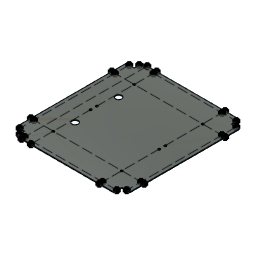
Hot Plate Mounting Plate (Autodesk Fusion 360 design; units mm, degrees)
Autodesk Fusion 360 part; units mm, degrees
sketch "Sketch1" plane through (0, 0, 0) normal (0, 0, 1) x (1, 0, 0) in component "Hot Plate Mounting Plate"
  line L0 (0, 0) -> (-182, 0) construction
  line L1 (-182, 0) -> (-182, -202) construction
  line L2 (-182, -202) -> (0, -202) construction
  line L3 (0, -202) -> (0, 0) construction
  line L4 (-91, -202) -> (-91, 0) construction
  line L5 (0, -101) -> (-182, -101) construction
  line L6 (-91, 0) -> (-13, 0)
  line L7 (-91, 0) -> (-169, 0)
  line L8 (-91, -202) -> (-13, -202)
  line L9 (-91, -202) -> (-169, -202)
  line L10 (0, -101) -> (0, -13)
  line L11 (0, -101) -> (0, -189)
  line L12 (-182, -101) -> (-182, -189)
  line L13 (-182, -101) -> (-182, -13)
  line L14 (-182, -13) -> (0, -13) construction
  line L15 (0, -189) -> (-182, -189) construction
  line L16 (-13, -202) -> (-13, 0) construction
  line L17 (-169, 0) -> (-169, -202) construction
  line L18 (0, -189) -> (-13, -189)
  line L19 (-13, -202) -> (-13, -189)
  line L20 (-169, -202) -> (-169, -189)
  line L21 (-182, -189) -> (-169, -189)
  line L22 (0, -13) -> (-13, -13)
  line L23 (-13, 0) -> (-13, -13)
  line L24 (-169, 0) -> (-169, -13)
  line L25 (-182, -13) -> (-169, -13)
  dimension "d1" = 182
  dimension "d2" = 202
  dimension "d3" = 78
  dimension "d4" = 78
  dimension "d5" = 78
  dimension "d6" = 78
  dimension "d7" = 88
  dimension "d8" = 88
  dimension "d9" = 88
  dimension "d10" = 88
  constraint horizontal L0
  constraint vertical L1
  constraint horizontal L2
  constraint vertical L3
  constraint coincident L0.start L3.end
  constraint midpoint L2 L4.start
  constraint midpoint L0 L4.end
  constraint midpoint L3 L5.start
  constraint midpoint L1 L5.end
  constraint perpendicular L4 L6
  constraint perpendicular L4 L7
  constraint perpendicular L4 L8
  constraint perpendicular L4 L9
  constraint perpendicular L5 L10
  constraint perpendicular L5 L11
  constraint perpendicular L5 L12
  constraint perpendicular L5 L13
  constraint coincident L15 L18.end
  constraint coincident L16 L18.end
  constraint coincident L15 L20.end
  constraint coincident L17 L20.end
  constraint coincident L14 L22.end
  constraint coincident L16 L22.end
  constraint coincident L14 L24.end
  constraint coincident L17 L24.end
  measures "d1" distance of L0.start L0.end
  measures "d2" distance of L0.start L2.end
  measures "d3" distance of L4.end L6.end
  measures "d4" distance of L4.end L7.end
  measures "d5" distance of L4.start L8.end
  measures "d6" distance of L4.start L9.end
  measures "d7" distance of L5.start L10.end
  measures "d8" distance of L5.start L11.end
  measures "d9" distance of L5.end L12.end
  measures "d10" distance of L5.end L13.end
extrude "Extrude1" add sketch "Sketch1" along normal blind 1 in component "Hot Plate Mounting Plate"
sketch "Sketch3" plane through (0, 0, 1) normal (0, 0, 1) x (-1, 0, 0) in component "Hot Plate Mounting Plate"
  line L0 (182, 13) -> (182, 189)
  line L1 (182, 189) -> (169, 189)
  line L2 (169, 189) -> (169, 202)
  line L3 (169, 202) -> (13, 202)
  line L4 (13, 202) -> (13, 189)
  line L5 (13, 189) -> (0, 189)
  line L6 (0, 189) -> (0, 13)
  line L7 (0, 13) -> (13, 13)
  line L8 (13, 13) -> (13, 0)
  line L9 (13, 0) -> (169, 0)
  line L10 (169, 0) -> (169, 13)
  line L11 (169, 13) -> (182, 13)
  line L12 (177, 13) -> (177, 189) construction
  line L13 (169, 5) -> (13, 5) construction
  line L14 (5, 13) -> (5, 189) construction
  line L15 (13, 197) -> (169, 197) construction
  line L16 (182, 36) -> (0, 36) construction
  line L17 (182, 166) -> (0, 166) construction
  line L18 (146, 0) -> (146, 202) construction
  line L19 (36, 0) -> (36, 202) construction
  circle A0 centre (146, 5) radius 1.75
  circle A1 centre (177, 36) radius 1.75
  circle A2 centre (177, 166) radius 1.75
  circle A3 centre (36, 197) radius 1.75
  circle A4 centre (5, 166) radius 1.75
  circle A5 centre (5, 36) radius 1.75
  circle A6 centre (36, 5) radius 1.75
  line L20 (161, 202) -> (161, 0) construction
  circle A7 centre (161, 197) radius 1.75
  dimension "d44" = 5
  dimension "d45" = 5
  dimension "d46" = 5
  dimension "d47" = 5
  dimension "d48" = 23
  dimension "d49" = 23
  dimension "d50" = 23
  dimension "d51" = 23
  dimension "d52" = 3.5
  dimension "d53" = 3.5
  dimension "d54" = 3.5
  dimension "d56" = 3.5
  dimension "d57" = 3.5
  dimension "d60" = 3.5
  dimension "d61" = 3.5
  dimension "d62" = 8
  dimension "d63" = 3.5
  constraint coincident L11 L12.start
  constraint coincident L1 L12.end
  constraint perpendicular L1 L12
  constraint coincident L10 L13.start
  constraint coincident L8 L13.end
  constraint perpendicular L8 L13
  constraint coincident L7 L14.start
  constraint coincident L5 L14.end
  constraint perpendicular L5 L14
  constraint coincident L4 L15.start
  constraint coincident L2 L15.end
  constraint perpendicular L2 L15
  constraint coincident L0 L16.start
  constraint coincident L6 L16.end
  constraint perpendicular L6 L16
  constraint coincident L0 L17.start
  constraint coincident L6 L17.end
  constraint perpendicular L6 L17
  constraint coincident L9 L18.start
  constraint perpendicular L9 L18
  constraint coincident L9 L19.start
  constraint coincident L3 L19.end
  constraint perpendicular L3 L19
  constraint coincident L13 A0.centre
  constraint coincident L18 A0.centre
  constraint coincident L16 A1.centre
  constraint coincident L12 A1.centre
  constraint coincident L17 A2.centre
  constraint coincident L12 A2.centre
  constraint coincident L3 L18.end
  constraint coincident L15 A3.centre
  constraint coincident L19 A3.centre
  constraint coincident L17 A4.centre
  constraint coincident L14 A4.centre
  constraint coincident L16 A5.centre
  constraint coincident L14 A5.centre
  constraint coincident L19 A6.centre
  constraint coincident L13 A6.centre
  constraint coincident L3 L20.start
  constraint coincident L9 L20.end
  constraint perpendicular L9 L20
  constraint coincident L15 A7.centre
  constraint coincident L20 A7.centre
  measures "d44" distance of L0 L12
  measures "d45" distance of L3 L15
  measures "d46" distance of L6 L14
  measures "d47" distance of L9 L13
  measures "d48" distance of L11 L16
  measures "d49" distance of L10 L18
  measures "d50" distance of L8 L19
  measures "d51" distance of L1 L17
  measures "d52" diameter of A0
  measures "d53" diameter of A1
  measures "d54" diameter of A2
  measures "d56" diameter of A3
  measures "d57" diameter of A4
  measures "d60" diameter of A5
  measures "d61" diameter of A6
  measures "d62" distance of L2 L20
  measures "d63" diameter of A7
extrude "Extrude3" cut sketch "Sketch3" against normal up to surface (1 mm away) contours A0 | A1 | A2 | A3 | A4 | A5 | A6 | A7 in component "Hot Plate Mounting Plate"
sketch "Sketch4" plane through (0, 0, 1) normal (0, 0, 1) x (-1, 0, 0) in component "Hot Plate Mounting Plate"
  circle A0 centre (5, 36) radius 1.75
  circle A1 centre (5, 166) radius 1.75
  circle A2 centre (177, 166) radius 1.75
  circle A3 centre (36, 5) radius 1.75
  circle A4 centre (146, 5) radius 1.75
  circle A5 centre (36, 197) radius 1.75
  circle A6 centre (177, 36) radius 1.75
  circle A7 centre (161, 197) radius 1.75
  line L0 (182, 13) -> (182, 189)
  line L1 (182, 189) -> (169, 189)
  line L2 (169, 189) -> (169, 202)
  line L3 (169, 202) -> (13, 202)
  line L4 (13, 202) -> (13, 189)
  line L5 (13, 189) -> (0, 189)
  line L6 (0, 189) -> (0, 13)
  line L7 (0, 13) -> (13, 13)
  line L8 (13, 13) -> (13, 0)
  line L9 (13, 0) -> (169, 0)
  line L10 (169, 0) -> (169, 13)
  line L11 (169, 13) -> (182, 13)
  line L12 (182, 101) -> (0, 101) construction
  line L13 (91, 0) -> (91, 202) construction
  line L14 (31, 31) -> (151, 31) construction
  line L15 (151, 31) -> (151, 171) construction
  line L16 (151, 171) -> (31, 171) construction
  line L17 (31, 171) -> (31, 31) construction
  line L18 (31, 31) -> (151, 171) construction
  line L19 (151, 31) -> (31, 171) construction
  line L20 (146, 31) -> (146, 171) construction
  line L21 (151, 36) -> (31, 36) construction
  line L22 (36, 31) -> (36, 171) construction
  line L23 (151, 166) -> (31, 166) construction
  circle A8 centre (146, 36) radius 1.75
  line L24 (151, 96) -> (31, 96) construction
  line L25 (151, 106) -> (31, 106) construction
  circle A9 centre (146, 96) radius 1.75
  circle A10 centre (36, 96) radius 1.75
  circle A11 centre (146, 106) radius 1.75
  circle A12 centre (36, 106) radius 1.75
  circle A13 centre (146, 166) radius 1.75
  circle A14 centre (36, 166) radius 1.75
  circle A15 centre (36, 36) radius 1.75
  line L26 (151, 66) -> (31, 66) construction
  line L27 (151, 136) -> (31, 136) construction
  line L28 (141, 31) -> (141, 171) construction
  circle A16 centre (141, 66) radius 5
  circle A17 centre (141, 136) radius 5
  point P0 (91, 101)
  dimension "d64" = 120
  dimension "d65" = 140
  dimension "d66" = 5
  dimension "d67" = 5
  dimension "d68" = 5
  dimension "d69" = 5
  dimension "d70" = 3.5
  dimension "d71" = 5
  dimension "d72" = 5
  dimension "d73" = 3.5
  dimension "d74" = 3.5
  dimension "d75" = 3.5
  dimension "d76" = 3.5
  dimension "d77" = 3.5
  dimension "d78" = 3.5
  dimension "d79" = 3.5
  dimension "d83" = 35
  dimension "d84" = 35
  dimension "d85" = 10
  dimension "d86" = 10
  dimension "d87" = 10
  constraint midpoint L0 L12.start
  constraint midpoint L6 L12.end
  constraint midpoint L9 L13.start
  constraint midpoint L3 L13.end
  constraint horizontal L14
  constraint perpendicular L14 L15
  constraint parallel L14 L16
  constraint parallel L15 L17
  constraint coincident L18 P0
  constraint coincident L19 P0
  constraint midpoint L12 P0
  constraint coincident L14 L20.start
  constraint coincident L16 L20.end
  constraint perpendicular L16 L20
  constraint coincident L15 L21.start
  constraint coincident L17 L21.end
  constraint perpendicular L17 L21
  constraint coincident L14 L22.start
  constraint coincident L16 L22.end
  constraint perpendicular L16 L22
  constraint coincident L15 L23.start
  constraint coincident L17 L23.end
  constraint perpendicular L17 L23
  constraint coincident L20 A8.centre
  constraint coincident L21 A8.centre
  constraint coincident L15 L24.start
  constraint coincident L17 L24.end
  constraint perpendicular L17 L24
  constraint coincident L15 L25.start
  constraint coincident L17 L25.end
  constraint perpendicular L17 L25
  constraint coincident L24 A9.centre
  constraint coincident L20 A9.centre
  constraint coincident L24 A10.centre
  constraint coincident L22 A10.centre
  constraint coincident L25 A11.centre
  constraint coincident L20 A11.centre
  constraint coincident L25 A12.centre
  constraint coincident L22 A12.centre
  constraint coincident L23 A13.centre
  constraint coincident L20 A13.centre
  constraint coincident L23 A14.centre
  constraint coincident L22 A14.centre
  constraint coincident L22 A15.centre
  constraint coincident L21 A15.centre
  constraint coincident L15 L26.start
  constraint coincident L17 L26.end
  constraint perpendicular L17 L26
  constraint coincident L15 L27.start
  constraint coincident L17 L27.end
  constraint perpendicular L17 L27
  constraint coincident L14 L28.start
  constraint coincident L16 L28.end
  constraint perpendicular L16 L28
  constraint coincident L26 A16.centre
  constraint coincident L28 A16.centre
  constraint coincident L27 A17.centre
  constraint coincident L28 A17.centre
  measures "d64" distance of L15.end L16.end
  measures "d65" distance of L14.end L15.end
  measures "d66" distance of L16 L23
  measures "d67" distance of L15 L20
  measures "d68" distance of L14 L21
  measures "d69" distance of L17 L22
  measures "d70" diameter of A8
  measures "d71" distance of L12 L24
  measures "d72" distance of L12 L25
  measures "d73" diameter of A9
  measures "d74" diameter of A10
  measures "d75" diameter of A11
  measures "d76" diameter of A12
  measures "d77" diameter of A13
  measures "d78" diameter of A14
  measures "d79" diameter of A15
  measures "d83" distance of L12 L26
  measures "d84" distance of L12 L27
  measures "d85" diameter of A16
  measures "d86" diameter of A17
  measures "d87" distance of L15 L28
extrude "Extrude4" cut sketch "Sketch4" against normal up to surface (1 mm away) contours A8 | A9 | A10 | A11 | A12 | A13 | A14 | A15 | A16 | A17 in component "Hot Plate Mounting Plate"
component "Hot Plate Mounting Plate" placed x (1, 0, 0) y (0, 1, 0) z (0, 0, 1) at (0, 0, 0)
